Autodesk Fusion 360 part; units mm, degrees
note: some values were not read from the file. Chosen so that the rebuilt part matches the saved one: which pieces of a blend or face edit are solid.
(part 4 of 4)
  arc A1155 (-328.0323, 104.3254) -> (-327.345, 105.0126) centre (-327.7718, 104.7521) ccw
  arc A1156 (-328.0323, 104.3254) -> (-328.1886, 104.3693) centre (-328.1885, 104.0696) ccw
  line L626 (-328.1886, 104.3693) -> (-329.0889, 104.3693)
  line L627 (-329.0889, 104.3693) -> (-329.9893, 104.3693)
  arc A1157 (-329.9893, 104.3693) -> (-330.1456, 104.3254) centre (-329.9893, 104.0693) ccw
  circle A1158 centre (-310.0389, 100.7893) radius 1.9939
  circle A1159 centre (-315.1189, 100.7893) radius 0.875
  circle A1160 centre (-306.2289, 98.2493) radius 1.5
  circle A1161 centre (-324.0089, 100.7893) radius 0.875
  circle A1162 centre (-329.0889, 100.7893) radius 1.9939
  circle A1163 centre (-334.1689, 100.7893) radius 0.875
  circle A1164 centre (-325.2789, 98.2493) radius 1.5
  circle A1165 centre (-343.0589, 100.7893) radius 0.875
  circle A1166 centre (-344.3289, 98.2493) radius 1.5
  arc A1167 (-349.8829, 105.0126) -> (-349.1956, 104.3254) centre (-349.4561, 104.7521) ccw
  arc A1168 (-349.8829, 105.0126) -> (-349.8389, 105.1689) centre (-350.1389, 105.1689) ccw
  line L628 (-349.8389, 105.1689) -> (-349.8389, 105.8693)
  line L629 (-349.8389, 105.8693) -> (-349.8389, 106.5696)
  arc A1169 (-349.8389, 106.5696) -> (-349.8829, 106.7259) centre (-350.1389, 106.5696) ccw
  arc A1170 (-349.1956, 107.4132) -> (-349.8829, 106.7259) centre (-349.4561, 106.9864) ccw
  arc A1171 (-349.1956, 107.4132) -> (-349.0393, 107.3693) centre (-349.0393, 107.6693) ccw
  line L630 (-349.0393, 107.3693) -> (-348.1389, 107.3693)
  line L631 (-348.1389, 107.3693) -> (-347.2386, 107.3693)
  arc A1172 (-347.2386, 107.3693) -> (-347.0823, 107.4132) centre (-347.2386, 107.6693) ccw
  arc A1173 (-346.395, 106.7259) -> (-347.0823, 107.4132) centre (-346.8218, 106.9864) ccw
  arc A1174 (-346.395, 106.7259) -> (-346.4389, 106.5696) centre (-346.1389, 106.5696) ccw
  line L632 (-346.4389, 106.5696) -> (-346.4389, 105.8693)
  line L633 (-346.4389, 105.8693) -> (-346.4389, 105.1689)
  arc A1175 (-346.4389, 105.1689) -> (-346.395, 105.0126) centre (-346.1389, 105.1689) ccw
  arc A1176 (-347.0823, 104.3254) -> (-346.395, 105.0126) centre (-346.8218, 104.7521) ccw
  arc A1177 (-347.0823, 104.3254) -> (-347.2386, 104.3693) centre (-347.2385, 104.0696) ccw
  line L634 (-347.2386, 104.3693) -> (-348.1389, 104.3693)
  line L635 (-348.1389, 104.3693) -> (-349.0393, 104.3693)
  arc A1178 (-349.0393, 104.3693) -> (-349.1956, 104.3254) centre (-349.0393, 104.0693) ccw
  arc A1179 (-368.9329, 105.0126) -> (-368.2456, 104.3254) centre (-368.5061, 104.7521) ccw
  arc A1180 (-368.9329, 105.0126) -> (-368.8889, 105.1689) centre (-369.1889, 105.1689) ccw
  line L636 (-368.8889, 105.1689) -> (-368.8889, 105.8693)
  line L637 (-368.8889, 105.8693) -> (-368.8889, 106.5696)
  arc A1181 (-368.8889, 106.5696) -> (-368.9329, 106.7259) centre (-369.1889, 106.5696) ccw
  arc A1182 (-368.2456, 107.4132) -> (-368.9329, 106.7259) centre (-368.5061, 106.9864) ccw
  arc A1183 (-368.2456, 107.4132) -> (-368.0893, 107.3693) centre (-368.0893, 107.6693) ccw
  line L638 (-368.0893, 107.3693) -> (-367.1889, 107.3693)
  line L639 (-367.1889, 107.3693) -> (-366.2886, 107.3693)
  arc A1184 (-366.2886, 107.3693) -> (-366.1323, 107.4132) centre (-366.2886, 107.6693) ccw
  arc A1185 (-365.445, 106.7259) -> (-366.1323, 107.4132) centre (-365.8718, 106.9864) ccw
  arc A1186 (-365.445, 106.7259) -> (-365.4889, 106.5696) centre (-365.1889, 106.5696) ccw
  line L640 (-365.4889, 106.5696) -> (-365.4889, 105.8693)
  line L641 (-365.4889, 105.8693) -> (-365.4889, 105.1689)
  arc A1187 (-365.4889, 105.1689) -> (-365.445, 105.0126) centre (-365.1889, 105.1689) ccw
  arc A1188 (-366.1323, 104.3254) -> (-365.445, 105.0126) centre (-365.8718, 104.7521) ccw
  arc A1189 (-366.1323, 104.3254) -> (-366.2886, 104.3693) centre (-366.2885, 104.0696) ccw
  line L642 (-366.2886, 104.3693) -> (-367.1889, 104.3693)
  line L643 (-367.1889, 104.3693) -> (-368.0893, 104.3693)
  arc A1190 (-368.0893, 104.3693) -> (-368.2456, 104.3254) centre (-368.0893, 104.0693) ccw
  circle A1191 centre (-348.1389, 100.7893) radius 1.9939
  circle A1192 centre (-353.2189, 100.7893) radius 0.875
  circle A1193 centre (-362.1089, 100.7893) radius 0.875
  circle A1194 centre (-363.3789, 98.2493) radius 1.5
  circle A1195 centre (-367.1889, 100.7893) radius 1.9939
  circle A1196 centre (-372.2689, 100.7893) radius 0.875
  circle A1197 centre (-381.1589, 100.7893) radius 0.875
  circle A1198 centre (-382.4289, 98.2493) radius 1.5
  arc A1199 (-397.5079, 124.0626) -> (-396.8206, 123.3754) centre (-397.0811, 123.8021) ccw
  arc A1200 (-397.5079, 124.0626) -> (-397.4639, 124.2189) centre (-397.7639, 124.2189) ccw
  line L644 (-397.4639, 124.2189) -> (-397.4639, 124.9193)
  line L645 (-397.4639, 124.9193) -> (-397.4639, 125.6196)
  arc A1201 (-397.4639, 125.6196) -> (-397.5079, 125.7759) centre (-397.7639, 125.6196) ccw
  arc A1202 (-396.8206, 126.4632) -> (-397.5079, 125.7759) centre (-397.0811, 126.0364) ccw
  arc A1203 (-396.8206, 126.4632) -> (-396.6643, 126.4193) centre (-396.6643, 126.7193) ccw
  line L646 (-396.6643, 126.4193) -> (-395.7639, 126.4193)
  line L647 (-395.7639, 126.4193) -> (-394.8636, 126.4193)
  arc A1204 (-394.8636, 126.4193) -> (-394.7073, 126.4632) centre (-394.8636, 126.7193) ccw
  arc A1205 (-394.02, 125.7759) -> (-394.7073, 126.4632) centre (-394.4468, 126.0364) ccw
  arc A1206 (-394.02, 125.7759) -> (-394.0639, 125.6196) centre (-393.7639, 125.6196) ccw
  line L648 (-394.0639, 125.6196) -> (-394.0639, 124.9193)
  line L649 (-394.0639, 124.9193) -> (-394.0639, 124.2189)
  arc A1207 (-394.0639, 124.2189) -> (-394.02, 124.0626) centre (-393.7639, 124.2189) ccw
  arc A1208 (-394.7073, 123.3754) -> (-394.02, 124.0626) centre (-394.4468, 123.8021) ccw
  arc A1209 (-394.7073, 123.3754) -> (-394.8636, 123.4193) centre (-394.8635, 123.1196) ccw
  line L650 (-394.8636, 123.4193) -> (-395.7639, 123.4193)
  line L651 (-395.7639, 123.4193) -> (-396.6643, 123.4193)
  arc A1210 (-396.6643, 123.4193) -> (-396.8206, 123.3754) centre (-396.6643, 123.1193) ccw
  arc A1211 (-421.3204, 124.0626) -> (-420.6331, 123.3754) centre (-420.8936, 123.8021) ccw
  arc A1212 (-421.3204, 124.0626) -> (-421.2764, 124.2189) centre (-421.5764, 124.2189) ccw
  line L652 (-421.2764, 124.2189) -> (-421.2764, 124.9193)
  line L653 (-421.2764, 124.9193) -> (-421.2764, 125.6196)
  arc A1213 (-421.2764, 125.6196) -> (-421.3204, 125.7759) centre (-421.5764, 125.6196) ccw
  arc A1214 (-420.6331, 126.4632) -> (-421.3204, 125.7759) centre (-420.8936, 126.0364) ccw
  arc A1215 (-420.6331, 126.4632) -> (-420.4768, 126.4193) centre (-420.4768, 126.7193) ccw
  line L654 (-420.4768, 126.4193) -> (-419.5764, 126.4193)
  line L655 (-419.5764, 126.4193) -> (-418.6761, 126.4193)
  arc A1216 (-418.6761, 126.4193) -> (-418.5198, 126.4632) centre (-418.6761, 126.7193) ccw
  arc A1217 (-417.8325, 125.7759) -> (-418.5198, 126.4632) centre (-418.2593, 126.0364) ccw
  arc A1218 (-417.8325, 125.7759) -> (-417.8764, 125.6196) centre (-417.5764, 125.6196) ccw
  line L656 (-417.8764, 125.6196) -> (-417.8764, 124.9193)
  line L657 (-417.8764, 124.9193) -> (-417.8764, 124.2189)
  arc A1219 (-417.8764, 124.2189) -> (-417.8325, 124.0626) centre (-417.5764, 124.2189) ccw
  arc A1220 (-418.5198, 123.3754) -> (-417.8325, 124.0626) centre (-418.2593, 123.8021) ccw
  arc A1221 (-418.5198, 123.3754) -> (-418.6761, 123.4193) centre (-418.676, 123.1196) ccw
  line L658 (-418.6761, 123.4193) -> (-419.5764, 123.4193)
  line L659 (-419.5764, 123.4193) -> (-420.4768, 123.4193)
  arc A1222 (-420.4768, 123.4193) -> (-420.6331, 123.3754) centre (-420.4768, 123.1193) ccw
  circle A1223 centre (-390.6839, 119.8393) radius 0.875
  circle A1224 centre (-391.9539, 117.2993) radius 1.5
  circle A1225 centre (-395.7639, 119.8393) radius 1.9939
  circle A1226 centre (-400.8439, 119.8393) radius 0.875
  circle A1227 centre (-398.3039, 114.7593) radius 1.5
  circle A1228 centre (-414.4964, 119.8393) radius 0.875
  circle A1229 centre (-419.5764, 119.8393) radius 1.9939
  circle A1230 centre (-415.7664, 117.2993) radius 1.5
  circle A1231 centre (-422.1164, 114.7593) radius 1.5
  arc A1232 (-454.6579, 124.0626) -> (-453.9706, 123.3754) centre (-454.2311, 123.8021) ccw
  arc A1233 (-454.6579, 124.0626) -> (-454.6139, 124.2189) centre (-454.9139, 124.2189) ccw
  line L660 (-454.6139, 124.2189) -> (-454.6139, 124.9193)
  line L661 (-454.6139, 124.9193) -> (-454.6139, 125.6196)
  arc A1234 (-454.6139, 125.6196) -> (-454.6579, 125.7759) centre (-454.9139, 125.6196) ccw
  arc A1235 (-453.9706, 126.4632) -> (-454.6579, 125.7759) centre (-454.2311, 126.0364) ccw
  arc A1236 (-453.9706, 126.4632) -> (-453.8143, 126.4193) centre (-453.8143, 126.7193) ccw
  line L662 (-453.8143, 126.4193) -> (-452.9139, 126.4193)
  line L663 (-452.9139, 126.4193) -> (-452.0136, 126.4193)
  arc A1237 (-452.0136, 126.4193) -> (-451.8573, 126.4632) centre (-452.0136, 126.7193) ccw
  arc A1238 (-451.17, 125.7759) -> (-451.8573, 126.4632) centre (-451.5968, 126.0364) ccw
  arc A1239 (-451.17, 125.7759) -> (-451.2139, 125.6196) centre (-450.9139, 125.6196) ccw
  line L664 (-451.2139, 125.6196) -> (-451.2139, 124.9193)
  line L665 (-451.2139, 124.9193) -> (-451.2139, 124.2189)
  arc A1240 (-451.2139, 124.2189) -> (-451.17, 124.0626) centre (-450.9139, 124.2189) ccw
  arc A1241 (-451.8573, 123.3754) -> (-451.17, 124.0626) centre (-451.5968, 123.8021) ccw
  arc A1242 (-451.8573, 123.3754) -> (-452.0136, 123.4193) centre (-452.0135, 123.1196) ccw
  line L666 (-452.0136, 123.4193) -> (-452.9139, 123.4193)
  line L667 (-452.9139, 123.4193) -> (-453.8143, 123.4193)
  arc A1243 (-453.8143, 123.4193) -> (-453.9706, 123.3754) centre (-453.8143, 123.1193) ccw
  circle A1244 centre (-424.6564, 119.8393) radius 0.875
  circle A1245 centre (-447.8339, 119.8393) radius 0.875
  circle A1246 centre (-452.9139, 119.8393) radius 1.9939
  circle A1247 centre (-449.1039, 117.2993) radius 1.5
  circle A1248 centre (-457.9939, 119.8393) radius 0.875
  circle A1249 centre (-455.4539, 114.7593) radius 1.5
  arc A1250 (-387.9829, 105.0126) -> (-387.2956, 104.3254) centre (-387.5561, 104.7521) ccw
  arc A1251 (-387.9829, 105.0126) -> (-387.9389, 105.1689) centre (-388.2389, 105.1689) ccw
  line L668 (-387.9389, 105.1689) -> (-387.9389, 105.8693)
  line L669 (-387.9389, 105.8693) -> (-387.9389, 106.5696)
  arc A1252 (-387.9389, 106.5696) -> (-387.9829, 106.7259) centre (-388.2389, 106.5696) ccw
  arc A1253 (-387.2956, 107.4132) -> (-387.9829, 106.7259) centre (-387.5561, 106.9864) ccw
  arc A1254 (-387.2956, 107.4132) -> (-387.1393, 107.3693) centre (-387.1393, 107.6693) ccw
  line L670 (-387.1393, 107.3693) -> (-386.2389, 107.3693)
  line L671 (-386.2389, 107.3693) -> (-385.3386, 107.3693)
  arc A1255 (-385.3386, 107.3693) -> (-385.1823, 107.4132) centre (-385.3386, 107.6693) ccw
  arc A1256 (-384.495, 106.7259) -> (-385.1823, 107.4132) centre (-384.9218, 106.9864) ccw
  arc A1257 (-384.495, 106.7259) -> (-384.5389, 106.5696) centre (-384.2389, 106.5696) ccw
  line L672 (-384.5389, 106.5696) -> (-384.5389, 105.8693)
  line L673 (-384.5389, 105.8693) -> (-384.5389, 105.1689)
  arc A1258 (-384.5389, 105.1689) -> (-384.495, 105.0126) centre (-384.2389, 105.1689) ccw
  arc A1259 (-385.1823, 104.3254) -> (-384.495, 105.0126) centre (-384.9218, 104.7521) ccw
  arc A1260 (-385.1823, 104.3254) -> (-385.3386, 104.3693) centre (-385.3385, 104.0696) ccw
  line L674 (-385.3386, 104.3693) -> (-386.2389, 104.3693)
  line L675 (-386.2389, 104.3693) -> (-387.1393, 104.3693)
  arc A1261 (-387.1393, 104.3693) -> (-387.2956, 104.3254) centre (-387.1393, 104.0693) ccw
  arc A1262 (-416.5579, 105.0126) -> (-415.8706, 104.3254) centre (-416.1311, 104.7521) ccw
  arc A1263 (-416.5579, 105.0126) -> (-416.5139, 105.1689) centre (-416.8139, 105.1689) ccw
  line L676 (-416.5139, 105.1689) -> (-416.5139, 105.8693)
  line L677 (-416.5139, 105.8693) -> (-416.5139, 106.5696)
  arc A1264 (-416.5139, 106.5696) -> (-416.5579, 106.7259) centre (-416.8139, 106.5696) ccw
  arc A1265 (-415.8706, 107.4132) -> (-416.5579, 106.7259) centre (-416.1311, 106.9864) ccw
  arc A1266 (-415.8706, 107.4132) -> (-415.7143, 107.3693) centre (-415.7143, 107.6693) ccw
  line L678 (-415.7143, 107.3693) -> (-414.8139, 107.3693)
  line L679 (-414.8139, 107.3693) -> (-413.9136, 107.3693)
  arc A1267 (-413.9136, 107.3693) -> (-413.7573, 107.4132) centre (-413.9136, 107.6693) ccw
  arc A1268 (-413.07, 106.7259) -> (-413.7573, 107.4132) centre (-413.4968, 106.9864) ccw
  arc A1269 (-413.07, 106.7259) -> (-413.1139, 106.5696) centre (-412.8139, 106.5696) ccw
  line L680 (-413.1139, 106.5696) -> (-413.1139, 105.8693)
  line L681 (-413.1139, 105.8693) -> (-413.1139, 105.1689)
  arc A1270 (-413.1139, 105.1689) -> (-413.07, 105.0126) centre (-412.8139, 105.1689) ccw
  arc A1271 (-413.7573, 104.3254) -> (-413.07, 105.0126) centre (-413.4968, 104.7521) ccw
  arc A1272 (-413.7573, 104.3254) -> (-413.9136, 104.3693) centre (-413.9135, 104.0696) ccw
  line L682 (-413.9136, 104.3693) -> (-414.8139, 104.3693)
  line L683 (-414.8139, 104.3693) -> (-415.7143, 104.3693)
  arc A1273 (-415.7143, 104.3693) -> (-415.8706, 104.3254) centre (-415.7143, 104.0693) ccw
  circle A1274 centre (-386.2389, 100.7893) radius 1.9939
  circle A1275 centre (-391.3189, 100.7893) radius 0.875
  circle A1276 centre (-409.7339, 100.7893) radius 0.875
  circle A1277 centre (-411.0039, 98.2493) radius 1.5
  circle A1278 centre (-414.8139, 100.7893) radius 1.9939
  circle A1279 centre (-419.8939, 100.7893) radius 0.875
  circle A1280 centre (-438.6264, 110.3143) radius 1.1
  arc A1281 (-452.2639, 105.6393) -> (-452.2639, 107.1393) centre (-452.2639, 106.3893) ccw
  line L684 (-452.2639, 105.6393) -> (-453.5639, 105.6393)
  arc A1282 (-453.5639, 107.1393) -> (-453.5639, 105.6393) centre (-453.5639, 106.3893) ccw
  line L685 (-453.5639, 107.1393) -> (-452.2639, 107.1393)
  circle A1283 centre (-445.9139, 103.2893) radius 0.5
  circle A1284 centre (-460.4139, 103.2893) radius 0.5
  circle A1285 centre (-452.9139, 100.7893) radius 1.05
  circle A1286 centre (-445.9139, 98.2893) radius 0.5
  arc A1287 (-457.1139, 99.9893) -> (-457.1139, 101.5893) centre (-457.1139, 100.7893) ccw
  line L686 (-457.1139, 99.9893) -> (-457.7139, 99.9893)
  arc A1288 (-457.7139, 101.5893) -> (-457.7139, 99.9893) centre (-457.7139, 100.7893) ccw
  line L687 (-457.7139, 101.5893) -> (-457.1139, 101.5893)
  circle A1289 centre (-460.4139, 100.7893) radius 0.5
  circle A1290 centre (-460.4139, 98.2893) radius 0.5
  circle A1291 centre (-312.5789, 95.7093) radius 1.5
  circle A1292 centre (-331.6289, 95.7093) radius 1.5
  arc A1293 (-321.3079, 81.2001) -> (-320.6206, 80.5129) centre (-320.8811, 80.9396) ccw
  arc A1294 (-321.3079, 81.2001) -> (-321.2639, 81.3564) centre (-321.5639, 81.3564) ccw
  line L688 (-321.2639, 81.3564) -> (-321.2639, 82.0568)
  line L689 (-321.2639, 82.0568) -> (-321.2639, 82.7571)
  arc A1295 (-321.2639, 82.7571) -> (-321.3079, 82.9134) centre (-321.5639, 82.7571) ccw
  arc A1296 (-320.6206, 83.6007) -> (-321.3079, 82.9134) centre (-320.8811, 83.1739) ccw
  arc A1297 (-320.6206, 83.6007) -> (-320.4643, 83.5568) centre (-320.4643, 83.8568) ccw
  line L690 (-320.4643, 83.5568) -> (-319.5639, 83.5568)
  line L691 (-319.5639, 83.5568) -> (-318.6636, 83.5568)
  arc A1298 (-318.6636, 83.5568) -> (-318.5073, 83.6007) centre (-318.6636, 83.8568) ccw
  arc A1299 (-317.82, 82.9134) -> (-318.5073, 83.6007) centre (-318.2468, 83.1739) ccw
  arc A1300 (-317.82, 82.9134) -> (-317.8639, 82.7571) centre (-317.5639, 82.7571) ccw
  line L692 (-317.8639, 82.7571) -> (-317.8639, 82.0568)
  line L693 (-317.8639, 82.0568) -> (-317.8639, 81.3564)
  arc A1301 (-317.8639, 81.3564) -> (-317.82, 81.2001) centre (-317.5639, 81.3564) ccw
  arc A1302 (-318.5073, 80.5129) -> (-317.82, 81.2001) centre (-318.2468, 80.9396) ccw
  arc A1303 (-318.5073, 80.5129) -> (-318.6636, 80.5568) centre (-318.6635, 80.2571) ccw
  line L694 (-318.6636, 80.5568) -> (-319.5639, 80.5568)
  line L695 (-319.5639, 80.5568) -> (-320.4643, 80.5568)
  arc A1304 (-320.4643, 80.5568) -> (-320.6206, 80.5129) centre (-320.4643, 80.2568) ccw
  circle A1305 centre (-331.4702, 88.883) radius 1.1
  arc A1306 (-345.1204, 81.2001) -> (-344.4331, 80.5129) centre (-344.6936, 80.9396) ccw
  arc A1307 (-345.1204, 81.2001) -> (-345.0764, 81.3564) centre (-345.3764, 81.3564) ccw
  line L696 (-345.0764, 81.3564) -> (-345.0764, 82.0568)
  line L697 (-345.0764, 82.0568) -> (-345.0764, 82.7571)
  arc A1308 (-345.0764, 82.7571) -> (-345.1204, 82.9134) centre (-345.3764, 82.7571) ccw
  arc A1309 (-344.4331, 83.6007) -> (-345.1204, 82.9134) centre (-344.6936, 83.1739) ccw
  arc A1310 (-344.4331, 83.6007) -> (-344.2768, 83.5568) centre (-344.2768, 83.8568) ccw
  line L698 (-344.2768, 83.5568) -> (-343.3764, 83.5568)
  line L699 (-343.3764, 83.5568) -> (-342.4761, 83.5568)
  arc A1311 (-342.4761, 83.5568) -> (-342.3198, 83.6007) centre (-342.4761, 83.8568) ccw
  arc A1312 (-341.6325, 82.9134) -> (-342.3198, 83.6007) centre (-342.0593, 83.1739) ccw
  arc A1313 (-341.6325, 82.9134) -> (-341.6764, 82.7571) centre (-341.3764, 82.7571) ccw
  line L700 (-341.6764, 82.7571) -> (-341.6764, 82.0568)
  line L701 (-341.6764, 82.0568) -> (-341.6764, 81.3564)
  arc A1314 (-341.6764, 81.3564) -> (-341.6325, 81.2001) centre (-341.3764, 81.3564) ccw
  arc A1315 (-342.3198, 80.5129) -> (-341.6325, 81.2001) centre (-342.0593, 80.9396) ccw
  arc A1316 (-342.3198, 80.5129) -> (-342.4761, 80.5568) centre (-342.476, 80.2571) ccw
  line L702 (-342.4761, 80.5568) -> (-343.3764, 80.5568)
  line L703 (-343.3764, 80.5568) -> (-344.2768, 80.5568)
  arc A1317 (-344.2768, 80.5568) -> (-344.4331, 80.5129) centre (-344.2768, 80.2568) ccw
  circle A1318 centre (-350.6789, 95.7093) radius 1.5
  circle A1319 centre (-369.7289, 95.7093) radius 1.5
  arc A1320 (-364.1704, 81.2001) -> (-363.4831, 80.5129) centre (-363.7436, 80.9396) ccw
  arc A1321 (-364.1704, 81.2001) -> (-364.1264, 81.3564) centre (-364.4264, 81.3564) ccw
  line L704 (-364.1264, 81.3564) -> (-364.1264, 82.0568)
  line L705 (-364.1264, 82.0568) -> (-364.1264, 82.7571)
  arc A1322 (-364.1264, 82.7571) -> (-364.1704, 82.9134) centre (-364.4264, 82.7571) ccw
  arc A1323 (-363.4831, 83.6007) -> (-364.1704, 82.9134) centre (-363.7436, 83.1739) ccw
  arc A1324 (-363.4831, 83.6007) -> (-363.3268, 83.5568) centre (-363.3268, 83.8568) ccw
  line L706 (-363.3268, 83.5568) -> (-362.4264, 83.5568)
  line L707 (-362.4264, 83.5568) -> (-361.5261, 83.5568)
  arc A1325 (-361.5261, 83.5568) -> (-361.3698, 83.6007) centre (-361.5261, 83.8568) ccw
  arc A1326 (-360.6825, 82.9134) -> (-361.3698, 83.6007) centre (-361.1093, 83.1739) ccw
  arc A1327 (-360.6825, 82.9134) -> (-360.7264, 82.7571) centre (-360.4264, 82.7571) ccw
  line L708 (-360.7264, 82.7571) -> (-360.7264, 82.0568)
  line L709 (-360.7264, 82.0568) -> (-360.7264, 81.3564)
  arc A1328 (-360.7264, 81.3564) -> (-360.6825, 81.2001) centre (-360.4264, 81.3564) ccw
  arc A1329 (-361.3698, 80.5129) -> (-360.6825, 81.2001) centre (-361.1093, 80.9396) ccw
  arc A1330 (-361.3698, 80.5129) -> (-361.5261, 80.5568) centre (-361.526, 80.2571) ccw
  line L710 (-361.5261, 80.5568) -> (-362.4264, 80.5568)
  line L711 (-362.4264, 80.5568) -> (-363.3268, 80.5568)
  arc A1331 (-363.3268, 80.5568) -> (-363.4831, 80.5129) centre (-363.3268, 80.2568) ccw
  arc A1332 (-383.2204, 81.2001) -> (-382.5331, 80.5129) centre (-382.7936, 80.9396) ccw
  arc A1333 (-383.2204, 81.2001) -> (-383.1764, 81.3564) centre (-383.4764, 81.3564) ccw
  line L712 (-383.1764, 81.3564) -> (-383.1764, 82.0568)
  line L713 (-383.1764, 82.0568) -> (-383.1764, 82.7571)
  arc A1334 (-383.1764, 82.7571) -> (-383.2204, 82.9134) centre (-383.4764, 82.7571) ccw
  arc A1335 (-382.5331, 83.6007) -> (-383.2204, 82.9134) centre (-382.7936, 83.1739) ccw
  arc A1336 (-382.5331, 83.6007) -> (-382.3768, 83.5568) centre (-382.3768, 83.8568) ccw
  line L714 (-382.3768, 83.5568) -> (-381.4764, 83.5568)
  line L715 (-381.4764, 83.5568) -> (-380.5761, 83.5568)
  arc A1337 (-380.5761, 83.5568) -> (-380.4198, 83.6007) centre (-380.5761, 83.8568) ccw
  arc A1338 (-379.7325, 82.9134) -> (-380.4198, 83.6007) centre (-380.1593, 83.1739) ccw
  arc A1339 (-379.7325, 82.9134) -> (-379.7764, 82.7571) centre (-379.4764, 82.7571) ccw
  line L716 (-379.7764, 82.7571) -> (-379.7764, 82.0568)
  line L717 (-379.7764, 82.0568) -> (-379.7764, 81.3564)
  arc A1340 (-379.7764, 81.3564) -> (-379.7325, 81.2001) centre (-379.4764, 81.3564) ccw
  arc A1341 (-380.4198, 80.5129) -> (-379.7325, 81.2001) centre (-380.1593, 80.9396) ccw
  arc A1342 (-380.4198, 80.5129) -> (-380.5761, 80.5568) centre (-380.576, 80.2571) ccw
  line L718 (-380.5761, 80.5568) -> (-381.4764, 80.5568)
  line L719 (-381.4764, 80.5568) -> (-382.3768, 80.5568)
  arc A1343 (-382.3768, 80.5568) -> (-382.5331, 80.5129) centre (-382.3768, 80.2568) ccw
  circle A1344 centre (-305.5939, 76.9768) radius 0.875
  circle A1345 centre (-314.4839, 76.9768) radius 0.875
  circle A1346 centre (-319.5639, 76.9768) radius 1.9939
  circle A1347 centre (-324.6439, 76.9768) radius 0.875
  circle A1348 centre (-315.7539, 74.4368) radius 1.5
  circle A1349 centre (-338.2964, 76.9768) radius 0.875
  circle A1350 centre (-343.3764, 76.9768) radius 1.9939
  circle A1351 centre (-339.5664, 74.4368) radius 1.5
  circle A1352 centre (-322.1039, 71.8968) radius 1.5
  circle A1353 centre (-331.4702, 67.4518) radius 1.1
  circle A1354 centre (-348.4564, 76.9768) radius 0.875
  circle A1355 centre (-357.3464, 76.9768) radius 0.875
  circle A1356 centre (-362.4264, 76.9768) radius 1.9939
  circle A1357 centre (-358.6164, 74.4368) radius 1.5
  circle A1358 centre (-367.5064, 76.9768) radius 0.875
  circle A1359 centre (-376.3964, 76.9768) radius 0.875
  circle A1360 centre (-381.4764, 76.9768) radius 1.9939
  circle A1361 centre (-377.6664, 74.4368) radius 1.5
  circle A1362 centre (-345.9164, 71.8968) radius 1.5
  circle A1363 centre (-364.9664, 71.8968) radius 1.5
  circle A1364 centre (-384.0164, 71.8968) radius 1.5
  circle A1365 centre (-388.7789, 95.7093) radius 1.5
  circle A1366 centre (-417.3539, 95.7093) radius 1.5
  circle A1367 centre (-414.7852, 90.5768) radius 0.5
  circle A1368 centre (-417.3252, 90.5768) radius 0.5
  circle A1369 centre (-419.8652, 90.5768) radius 0.5
  circle A1370 centre (-422.4052, 90.5768) radius 0.5
  arc A1371 (-402.2704, 81.2001) -> (-401.5831, 80.5129) centre (-401.8436, 80.9396) ccw
  arc A1372 (-402.2704, 81.2001) -> (-402.2264, 81.3564) centre (-402.5264, 81.3564) ccw
  line L720 (-402.2264, 81.3564) -> (-402.2264, 82.0568)
  line L721 (-402.2264, 82.0568) -> (-402.2264, 82.7571)
  arc A1373 (-402.2264, 82.7571) -> (-402.2704, 82.9134) centre (-402.5264, 82.7571) ccw
  arc A1374 (-401.5831, 83.6007) -> (-402.2704, 82.9134) centre (-401.8436, 83.1739) ccw
  arc A1375 (-401.5831, 83.6007) -> (-401.4268, 83.5568) centre (-401.4268, 83.8568) ccw
  line L722 (-401.4268, 83.5568) -> (-400.5264, 83.5568)
  line L723 (-400.5264, 83.5568) -> (-399.6261, 83.5568)
  arc A1376 (-399.6261, 83.5568) -> (-399.4698, 83.6007) centre (-399.6261, 83.8568) ccw
  arc A1377 (-398.7825, 82.9134) -> (-399.4698, 83.6007) centre (-399.2093, 83.1739) ccw
  arc A1378 (-398.7825, 82.9134) -> (-398.8264, 82.7571) centre (-398.5264, 82.7571) ccw
  line L724 (-398.8264, 82.7571) -> (-398.8264, 82.0568)
  line L725 (-398.8264, 82.0568) -> (-398.8264, 81.3564)
  arc A1379 (-398.8264, 81.3564) -> (-398.7825, 81.2001) centre (-398.5264, 81.3564) ccw
  arc A1380 (-399.4698, 80.5129) -> (-398.7825, 81.2001) centre (-399.2093, 80.9396) ccw
  arc A1381 (-399.4698, 80.5129) -> (-399.6261, 80.5568) centre (-399.626, 80.2571) ccw
  line L726 (-399.6261, 80.5568) -> (-400.5264, 80.5568)
  line L727 (-400.5264, 80.5568) -> (-401.4268, 80.5568)
  arc A1382 (-401.4268, 80.5568) -> (-401.5831, 80.5129) centre (-401.4268, 80.2568) ccw
  circle A1383 centre (-424.9452, 90.5768) radius 0.5
  circle A1384 centre (-427.4852, 90.5768) radius 0.5
  circle A1385 centre (-430.0252, 90.5768) radius 0.5
  circle A1386 centre (-432.5652, 90.5768) radius 0.5
  circle A1387 centre (-435.1052, 90.5768) radius 0.5
  circle A1388 centre (-437.6452, 90.5768) radius 0.5
  circle A1389 centre (-440.1852, 90.5768) radius 0.5
  circle A1390 centre (-442.7252, 90.5768) radius 0.5
  arc A1391 (-452.2639, 94.4393) -> (-452.2639, 95.9393) centre (-452.2639, 95.1893) ccw
  line L728 (-452.2639, 94.4393) -> (-453.5639, 94.4393)
  arc A1392 (-453.5639, 95.9393) -> (-453.5639, 94.4393) centre (-453.5639, 95.1893) ccw
  line L729 (-453.5639, 95.9393) -> (-452.2639, 95.9393)
  circle A1393 centre (-445.2652, 90.5768) radius 0.5
  circle A1394 centre (-447.8052, 90.5768) radius 0.5
  circle A1395 centre (-450.3452, 90.5768) radius 0.5
  circle A1396 centre (-452.8852, 90.5768) radius 0.5
  circle A1397 centre (-455.4252, 90.5768) radius 0.5
  circle A1398 centre (-457.9652, 90.5768) radius 0.5
  circle A1399 centre (-460.5052, 90.5768) radius 0.5
  circle A1400 centre (-463.0452, 90.5768) radius 0.5
  circle A1401 centre (-462.8152, 84.2368) radius 0.5
  circle A1402 centre (-462.8152, 81.6968) radius 0.5
  circle A1403 centre (-386.5564, 76.9768) radius 0.875
  circle A1404 centre (-395.4464, 76.9768) radius 0.875
  circle A1405 centre (-400.5264, 76.9768) radius 1.9939
  circle A1406 centre (-396.7164, 74.4368) radius 1.5
  circle A1407 centre (-405.6064, 76.9768) radius 0.875
  circle A1408 centre (-403.0664, 71.8968) radius 1.5
  circle A1409 centre (-414.7852, 72.8068) radius 0.5
  circle A1410 centre (-417.3252, 72.7968) radius 0.5
  circle A1411 centre (-419.8652, 72.7968) radius 0.5
  circle A1412 centre (-422.4052, 72.7968) radius 0.5
  circle A1413 centre (-410.0514, 67.4518) radius 1.1
  circle A1414 centre (-462.8152, 79.1568) radius 0.5
  circle A1415 centre (-424.9452, 72.7968) radius 0.5
  circle A1416 centre (-427.4852, 72.7968) radius 0.5
  circle A1417 centre (-430.0252, 72.7968) radius 0.5
  circle A1418 centre (-432.5652, 72.7968) radius 0.5
  circle A1419 centre (-435.1052, 72.7968) radius 0.5
  circle A1420 centre (-437.6452, 72.7968) radius 0.5
  circle A1421 centre (-440.1852, 72.7968) radius 0.5
  circle A1422 centre (-442.7252, 72.7968) radius 0.5
  circle A1423 centre (-442.7902, 70.7393) radius 0.2
  circle A1424 centre (-443.6502, 70.7393) radius 0.2
  arc A1425 (-441.8002, 69.5893) -> (-441.1002, 69.5893) centre (-441.4502, 69.5893) ccw
  line L730 (-441.8002, 69.5893) -> (-441.8002, 70.8893)
  arc A1426 (-441.1002, 70.8893) -> (-441.8002, 70.8893) centre (-441.4502, 70.8893) ccw
  line L731 (-441.1002, 70.8893) -> (-441.1002, 69.5893)
  circle A1427 centre (-442.7902, 69.3893) radius 0.2
  circle A1428 centre (-443.6502, 69.3893) radius 0.2
  arc A1429 (-441.8002, 65.6493) -> (-441.1002, 65.6493) centre (-441.4502, 65.6493) ccw
  line L732 (-441.8002, 65.6493) -> (-441.8002, 66.5493)
  arc A1430 (-441.1002, 66.5493) -> (-441.8002, 66.5493) centre (-441.4502, 66.5493) ccw
  line L733 (-441.1002, 66.5493) -> (-441.1002, 65.6493)
  circle A1431 centre (-445.2652, 72.7968) radius 0.5
  circle A1432 centre (-447.8052, 72.7968) radius 0.5
  circle A1433 centre (-450.3452, 72.7968) radius 0.5
  circle A1434 centre (-452.8852, 72.7968) radius 0.5
  circle A1435 centre (-444.4902, 70.7393) radius 0.2
  circle A1436 centre (-445.3502, 70.7393) radius 0.2
  circle A1437 centre (-446.1902, 70.7393) radius 0.2
  circle A1438 centre (-447.0502, 70.7393) radius 0.2
  circle A1439 centre (-447.8902, 70.7393) radius 0.2
  circle A1440 centre (-444.4902, 69.3893) radius 0.2
  circle A1441 centre (-445.3502, 69.3893) radius 0.2
  circle A1442 centre (-446.1902, 69.3893) radius 0.2
  circle A1443 centre (-447.0502, 69.3893) radius 0.2
  circle A1444 centre (-447.8902, 69.3893) radius 0.2
  circle A1445 centre (-448.7502, 70.7393) radius 0.2
  arc A1446 (-450.4402, 69.5893) -> (-449.7402, 69.5893) centre (-450.0902, 69.5893) ccw
  line L734 (-450.4402, 69.5893) -> (-450.4402, 70.8893)
  arc A1447 (-449.7402, 70.8893) -> (-450.4402, 70.8893) centre (-450.0902, 70.8893) ccw
  line L735 (-449.7402, 70.8893) -> (-449.7402, 69.5893)
  circle A1448 centre (-448.7502, 69.3893) radius 0.2
  circle A1449 centre (-455.4252, 72.7968) radius 0.5
  circle A1450 centre (-457.9652, 72.7968) radius 0.5
  circle A1451 centre (-460.5052, 72.7968) radius 0.5
  circle A1452 centre (-463.0452, 72.7968) radius 0.5
  arc A1453 (-450.4402, 65.6493) -> (-449.7402, 65.6493) centre (-450.0902, 65.6493) ccw
  line L736 (-450.4402, 65.6493) -> (-450.4402, 66.5493)
  arc A1454 (-449.7402, 66.5493) -> (-450.4402, 66.5493) centre (-450.0902, 66.5493) ccw
  line L737 (-449.7402, 66.5493) -> (-449.7402, 65.6493)
  circle A1455 centre (-454.0252, 67.4518) radius 0.45
  circle A1456 centre (-456.5652, 67.4518) radius 0.45
  circle A1457 centre (-462.4389, 67.4518) radius 1.1
  circle A1458 centre (-169.5452, 67.4518) radius 1.1
  circle A1459 centre (-148.1139, 67.4518) radius 1.1
  circle A1460 centre (-169.5452, 88.883) radius 1.1
  circle A1461 centre (-148.1139, 129.3643) radius 1.1
  circle A1462 centre (-148.1139, 191.2768) radius 1.1
  circle A1463 centre (-245.7452, 191.2768) radius 1.1
  circle A1464 centre (-326.7077, 191.2768) radius 1.1
  circle A1465 centre (-462.4389, 191.2768) radius 1.1
  circle A1466 centre (-438.6264, 148.4143) radius 1.1
  circle A1467 centre (-462.4389, 129.3643) radius 1.1
  circle A1468 centre (-438.6264, 110.3143) radius 1.1
  circle A1469 centre (-462.4389, 67.4518) radius 1.1
  circle A1470 centre (-410.0514, 67.4518) radius 1.1
  circle A1471 centre (-331.4702, 88.883) radius 1.1
  circle A1472 centre (-331.4702, 67.4518) radius 1.1
  circle A1473 centre (-250.5077, 88.883) radius 1.1
  circle A1474 centre (-250.5077, 67.4518) radius 1.1
  constraint concentric A981 A1458
  constraint concentric A979 A1459
  constraint concentric A931 A1460
  constraint concentric A186 A1461
  constraint concentric A0 A1462
  constraint concentric A88 A1463
  constraint concentric A324 A1464
  constraint concentric A452 A1465
  constraint concentric A616 A1466
  constraint concentric A652 A1467
  constraint concentric A1280 A1468
  constraint concentric A1457 A1469
  constraint concentric A1413 A1470
  constraint concentric A1305 A1471
  constraint concentric A1353 A1472
  constraint concentric A1006 A1473
  constraint concentric A1054 A1474
extrude "Extrude5" cut sketch "Sketch2" against normal blind 93 contours A0 A1462 | A88 A1463 | A186 A1461 | A324 A1464 | A452 A1465 | A616 A1466 | A652 A1467 | A931 A1460 | A979 A1459 | A981 A1458 | A1006 A1473 | A1054 A1474 | A1280 A1468 | A1305 A1471 | A1353 A1472 | A1413 A1470 | A1457 A1469 bodies 3
move_body "Move1" bodies 2 3 to x (1, 0, 0) y (0, 1, 0) z (0, 0, 1) at (0, 0, -10)
move_body "Move2" bodies 2 3 to x (1, 0, 0) y (0, 1, 0) z (0, 0, 1) at (0, 0, 7.5)
extrude "Extrude6" add sketch "Sketch1" along normal blind 2.5 and the other way blind 1 contours L256 L257 L258 L259 L260 L261 L262 L263 L264 L265 L266 L267 L268 L269 L270 L271 L272 L273 L274 L275 L276 L277 L278 L279 L280 L281 L282 L283 L284 L285 L286 L287 L288 L289 L290 L291 L292 L293 L294 L295 L296 L297 L298 L299 L300 L301 L302 L303 L304 L305 L306 L307 L308 L309 L310 L311 L312 L313 L314 L315 L316 L317 L318 L319 L320 L321 L322 L323 L324 L325 L326 L327 L328 L329 L330 L331 L332 L333 L334 L335 L336 L337 L338 L339 bodies 2
extrude "Extrude9" add 1 faces at (227.3668, -85.3783, -2.5) along direction (0, 0, -1) blind 15 on bodies 3 bodies 3
draft "Draft2" angle -5 neutral plane through (0, 0, 0) pull (0, 1, 0) 1 faces at (227.3668, -85.3783, -1) on bodies 3
move_body "Move3" bodies 3 to x (1, 0, 0) y (0, 1, 0) z (0, 0, 1) at (0, 0, 15)
hidden bodies 1
